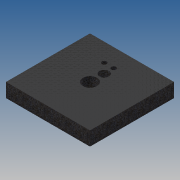
# Autodesk Inventor part: plinth
Saved by Autodesk Inventor 2014 SP1 (Build 180222100, 222)
## iProperties
Created: 2014-03-11
Part Number: plinth
Material: Concrete
Document SubType Name: Modeling
Designer: Dave
Density: 2.40731 g/cm^3
Appearance: Exposed Aggregate - Coarse
Mass: 77996.9 g
Surface Area: 17640 cm^2
Volume: 32400 cm^3
Author: Dave
Autodesk Inventor part; units mm, degrees
ref_plane "YZ Plane" through (0, 0, 0) normal (1, 0, 0) x (0, 1, 0)
ref_plane "XZ Plane" through (0, 0, 0) normal (0, 1, 0) x (-1, 0, 0)
ref_plane "XY Plane" through (0, 0, 0) normal (0, 0, 1) x (1, 0, 0)
sketch "Sketch1" plane through (0, 0, 0) normal (0, 1, 0) x (-1, 0, 0)
  line L0 (0, 0) -> (900, 0)
  line L1 (900, 0) -> (900, 900)
  line L2 (900, 900) -> (0, 900)
  line L3 (0, 900) -> (0, 0)
  dimension "d0" = 900
  dimension "d1" = 900
  constraints: 8 end point, 2 parallel, 1 horizontal, 1 perpendicular
  measures "d0" distance of L2.end L1.end
  measures "d1" distance of L2.end L0.start
extrude "base" add sketch "Sketch1" along normal blind 150
sketch "Sketch2" plane through (0, 150, 0) normal (0, 1, 0) x (1, 0, 0)
  circle A0 centre (-450, -450) radius 76.2
  dimension "d4" = 152.4
  constraints: 1 centre point
  measures "d4" diameter of A0
extrude "air" cut sketch "Sketch2" against normal through all
sketch "Sketch3" plane through (0, 150, 0) normal (0, 1, 0) x (1, 0, 0)
  circle A0 centre (-450, -450) radius 76.2 projected
  circle A1 centre (-450, -196) radius 25.4
  dimension "d7" = 50.8
  dimension "d8" = 254
  constraints: 1 centre point
  measures "d7" diameter of A1
  measures "d8" distance of A1.centre A0.centre
extrude "power" cut sketch "Sketch3" against normal blind 254 contours A1
sketch "Sketch5" plane through (0, 150, 0) normal (0, 1, 0) x (1, 0, 0)
  circle A0 centre (-450, -196) radius 25.4 projected
  circle A1 centre (-551.6, -196) radius 25.4
  dimension "d20" = 50.8
  dimension "d21" = 101.6
  constraints: 1 centre point
  measures "d20" diameter of A1
  measures "d21" distance of A1.centre A0.centre
hole "power2" at (-551.6, 150, 196) direction (0, -1, 0) diameter 50.8 end through all
sketch "Sketch4" plane through (0, 150, 0) normal (0, 1, 0) x (1, 0, 0)
  circle A0 centre (-450, -196) radius 25.4 projected
  circle A1 centre (-450, -450) radius 76.2 projected
  line L0 (0, -900) -> (0, 0) projected
  circle A2 centre (-450, -297.6) radius 25.4
  line L1 (-450, -196) -> (-450, -450) construction
  dimension "d11" = 50.8
  dimension "d12" = 101.6
  constraints: 2 end point, 1 centre point, 1 parallel
  measures "d11" diameter of A2
  measures "d12" distance of A2.centre L1.start
hole "fibre" at (-450, 150, 297.6) direction (0, -1, 0) diameter 101.6 end through all
body "Solid1"
